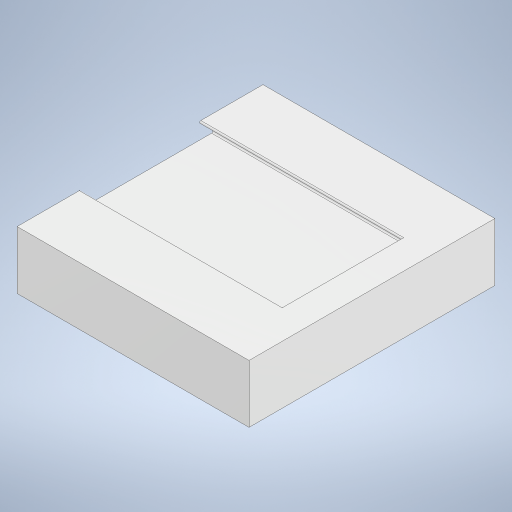
# Autodesk Inventor part: connector_part
Saved by Autodesk Inventor 2023 (Build 270158000, 158)
## iProperties
Created: 2022-06-20
Part Number: connector_part
Material: FormLabs Resin
Document SubType Name: Modeling
Designer: dennis
Density: 1.06 g/cm^3
Appearance: Smooth - White(1)
Author: dennis
Autodesk Inventor part; units mm, degrees
ref_plane "XZ Plane" through (0, 0, 0) normal (0, 1, 0) x (-1, 0, 0)
ref_plane "XY Plane" through (0, 0, 0) normal (0, 0, 1) x (1, 0, 0)
sketch "Sketch1" plane through (0, 0, 0) normal (0, 1, 0) x (-1, 0, 0)
  line L0 (20.00682, 15) -> (-19.99318, 15)
  line L1 (-19.99318, 15) -> (-19.99318, -15)
  line L2 (-19.99318, -15) -> (20.00682, -15)
  line L3 (20.00682, -15) -> (20.00682, 15)
  line L4 (-19.99318, 0) -> (-9.99318, 0)
  line L5 (-9.99318, 0) -> (-9.99318, -15)
  line L6 (-9.99318, 15) -> (-9.99318, 0)
  line L7 (-19.99318, -15) -> (-14.99318, -15)
  arc A0 (-17.49318, -15) -> (-12.49318, -15) centre (-14.99318, -12.194216) ccw
  line L8 (20.00682, -21.2) -> (-19.99318, -21.2)
  line L9 (-19.99318, -21.2) -> (-19.99318, 21.2)
  line L10 (-19.99318, 21.2) -> (20.00682, 21.2)
  line L11 (20.00682, 21.2) -> (20.00682, -21.2)
  line L12 (20.00682, -15) -> (20.00682, -21.2)
  line L13 (20.00682, -21.2) -> (13.80682, -21.2)
  line L14 (20.00682, 0) -> (-19.99318, 0)
  line L15 (15.40682, -21.2) -> (15.40682, -16.6)
  line L16 (15.40682, -16.6) -> (20.00682, -16.6)
  circle A1 centre (15.40682, -16.6) radius 1.6
  line L17 (0.00682, -15) -> (0.00682, 15)
  circle A2 centre (-15.39318, -16.6) radius 1.6
  circle A3 centre (15.40682, 16.6) radius 1.6
  circle A4 centre (-15.39318, 16.6) radius 1.6
  point P0 (20.00682, -1.119224)
  point P1 (-19.99318, 15)
  dimension "d6" = 40
  dimension "d7" = 30
  dimension "d17" = 10
  dimension "d25" = 5
  dimension "d33" = 42.4
  dimension "d34" = 6.2
  dimension "d35" = 6.2
  dimension "d37" = 4.6
  dimension "d38" = 3.2
  constraints: 36 end point, 8 point on line, 7 perpendicular, 5 centre point, 4 midpoint, 4 parallel, 3 horizontal, 3 symmetric about line, 2 point on circle, 1 coincident, 3 other
  measures "d6" distance of L2.end L1.end
  measures "d7" distance of L1.end L0.end
  measures "d17" distance of L4.start L4.end
  measures "d25" distance of A0.start A0.end
  measures "d33" distance of L8.end L9.end
  measures "d34" distance of L2.end L8.start
  measures "d35" distance of L8.start L13.end
  measures "d37" distance of L15.start L15.end
  measures "d38" diameter of A1
extrude "Extrusion1" add sketch "Sketch1" along normal blind 10 contours L17 L14 L6 L0 | L0 L3 L14 L17 | L6 L4 L1 L0 | L17 L2 L5 L14 | L14 L3 L2 L17 | L5 L2 L1 L4
sketch "Sketch2" plane through (19.99318, 0, 15) normal (1, 0, 0) x (0, 0, -1)
  line L0 (0, 10) -> (30, 10)
  line L1 (0, 0) -> (30, 0)
  line L2 (30, 10) -> (25, 10)
  line L3 (25, 10) -> (29.038687, 10) construction
  line L4 (25, 10) -> (27.828427, 7.171573)
  line L5 (25, 10) -> (29, 10) construction
  line L6 (15, 7.171573) -> (27.828427, 7.171573)
  line L7 (15, 10) -> (15, 7.171573)
  line L8 (5, 10) -> (2.171573, 7.171573)
  line L9 (15, 7.171573) -> (2.171573, 7.171573)
  point P0 (15, 0)
  point P1 (15, 0)
  dimension "d10" = 10
  dimension "d11" = 5
  dimension "d13" = 4
  dimension "d14" = 45
  constraints: 16 end point, 3 horizontal, 2 midpoint, 2 symmetric about line, 1 equal length, 1 point on line, 1 vertical
  measures "d10" distance from line of L0 point (15, 0)
  measures "d11" distance of L0.end L2.end
  measures "d13" distance of L2.end L4.end
  measures "d14" angle of L4 L5
extrude "Extrusion2" cut sketch "Sketch2" against normal blind 35
sketch "Skizze7" plane through (19.99318, 0, 15) normal (1, 0, 0) x (0, 0, -1)
  line L0 (25, 10) -> (27.828427, 7.171573)
  line L1 (26.414214, 8.585786) -> (27.914214, 8.585786) construction
  arc A0 (27.164214, 7.835786) -> (25.535463, 9.464537) centre (25.670285, 7.970608) ccw
  line L2 (5, 10) -> (25, 10)
  line L3 (15, 10) -> (15, 7.171573)
  line L4 (27.828427, 7.171573) -> (2.171573, 7.171573)
  arc A1 (4.464537, 9.464537) -> (2.835786, 7.835786) centre (4.329715, 7.970608) ccw
  point P0 (15, 0)
  dimension "d24" = 1.5
  constraints: 4 end point, 4 point on circle, 3 midpoint, 3 symmetric about line, 2 centre point, 2 point on line, 1 horizontal, 1 other
  measures "d24" radius of A0
ref_plane "Arbeitsebene1" through (17.5, 0, 0) normal (1, 0, 0) x (0, 1, 0)
extrude "Extrusion3" cut sketch "Skizze7" against normal blind 5 from surface at -2.49318 contours A0 L0
mirror "Spiegeln1" about plane through (0, 0, 0) normal (0, 0, 1) of "Extrusion3"
fillet "Rundung1" radius 2 1 edges at (17.5, 8.6502, -11.3498)
mirror "Spiegeln2" about plane through (0, 0, 0) normal (0, 0, 1) of "Rundung1"
sketch "Skizze8" plane through (19.99318, 0, 15) normal (1, 0, 0) x (0, 0, -1)
  line L0 (2.171573, 7.171573) -> (5, 10)
  line L1 (5, 10) -> (2.171573, 7.171573)
  line L2 (25, 10) -> (27.828427, 7.171573)
  line L3 (2.171573, 7.171573) -> (27.828427, 7.171573)
  line L4 (27.828427, 7.171573) -> (25, 10)
  line L5 (25, 10) -> (5, 10)
  line L6 (27.345584, 7.371573) -> (2.654416, 7.371573)
  line L7 (2.654416, 7.371573) -> (5.082843, 9.8)
  line L8 (24.917157, 9.8) -> (27.345584, 7.371573)
  line L9 (25, 10) -> (30, 10)
  line L10 (5, 10) -> (25, 10)
  line L11 (30, 10) -> (25, 10)
  line L12 (24.917157, 9.8) -> (24.917157, 10.2)
  line L13 (24.917157, 10.2) -> (30, 10.2)
  line L14 (15, 10) -> (15, 7.371573)
  line L15 (5.082843, 9.8) -> (5.082843, 10.2)
  line L16 (5.082843, 10.2) -> (0, 10.2)
  point P0 (15, 0)
  dimension "d30" = 0.2
  constraints: 26 end point, 3 collinear, 2 midpoint, 2 symmetric about line, 1 horizontal, 1 perpendicular, 1 vertical, 1 other
  measures "d30" distance between parallel lines of L3 L6
fillet "Rundung2" radius 0.2 4 edges at (2.4932, 7.1716, -12.8284) (2.4932, 7.1716, 12.8284) (2.4932, 10, 10) (2.4932, 10, -10)
extrude "Extrusion4" add sketch "Sketch1" along normal blind 10 contours A3 | A4 | L0 L9 L10 L11
mirror "Spiegeln3" about plane through (0, 0, 0) normal (0, 0, 1) of "Extrusion4"
extrude "Extrusion5" cut sketch "Sketch1" along normal blind 8 contours A3 | A4
mirror "Spiegeln4" about plane through (0, 0, 0) normal (0, 0, 1) of "Extrusion5"
move or copy body "Move Body1" bodies to move or copy 1 copy no rotation origin (0, 0, 0) rotation axis (0, 1, 0) rotation angle 180 translate (-40.01364, 0, 42.4)
move or copy body "Move Body2" bodies to move or copy 1 copy no translate (40, 0, -40)
ref_plane "Arbeitsebene2" through (0, 0, 0) normal (0, 0, 1) x (1, 0, 0)
body "Solid1"
